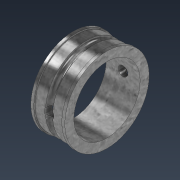
# Autodesk Inventor part: Łożysko wału korbowego 2
Saved by Autodesk Inventor 2022 (Build 260153000, 153)
## iProperties
Created: 2023-05-20
Part Number: Łożysko wału korbowego 2
Material: Generic
Document SubType Name: Modeling
Designer: wikto
Density: 1 g/cm^3
Appearance: Steel Galvanized
Author: wikto
Autodesk Inventor part; units mm, degrees
ref_plane "YZ Plane" through (0, 0, 0) normal (1, 0, 0) x (0, 1, 0)
ref_plane "XZ Plane" through (0, 0, 0) normal (0, 1, 0) x (-1, 0, 0)
ref_plane "XY Plane" through (0, 0, 0) normal (0, 0, 1) x (1, 0, 0)
sketch "Sketch1" plane through (0, 0, 0) normal (0, 0, 1) x (1, 0, 0)
  line L0 (-50, 0) -> (50, 0)
  line L1 (-14.086, 27.5) -> (-14.086, 35)
  line L2 (-14.086, 27.5) -> (14.086, 27.5)
  line L3 (14.086, 27.5) -> (14.086, 35)
  arc A0 (-3, 34) -> (3, 34) centre (0, 34) ccw
  line L4 (-14.086, 35) -> (-11.586, 35)
  line L5 (-11.586, 35) -> (-11.586, 34)
  line L6 (-11.586, 34) -> (-3, 34)
  line L7 (14.086, 35) -> (11.586, 35)
  line L8 (11.586, 35) -> (11.586, 34)
  line L9 (11.586, 34) -> (3, 34)
  point P0 (0, 0)
  point P1 (0, 0)
  point P2 (0, 27.5)
  dimension "d0" = 100
  dimension "d1" = 3
  dimension "d3" = 55
  dimension "d4" = 28.172
  dimension "d9" = 2.5
  dimension "d10" = 1
  dimension "d11" = 70
  constraints: 20 end point, 5 perpendicular, 4 horizontal, 2 equal length, 2 horizontal alignment, 2 midpoint, 2 point on circle, 2 vertical alignment, 1 centre point, 1 coincident, 1 vertical
  measures "d0" distance of L0.start L0.end
  measures "d1" radius of A0
  measures "d3" diameter of L2 L0
  measures "d4" distance between parallel lines of L3 L1
  measures "d9" distance of L3.end L7.end
  measures "d10" distance between parallel lines of L6 L4
  measures "d11" diameter of L7 L0
revolve "Revolution1" add sketch "Sketch1" angle 360 about axis through (-50, 0, 0) along (1, 0, 0)
sketch "Sketch2" plane through (0, 0, 0) normal (0, 0, 1) x (1, 0, 0)
  circle A0 centre (0, 0) radius 4
  dimension "d6" = 8
  constraints: 1 centre point, 1 coincident
  measures "d6" diameter of A0
extrude "Extrusion1" cut sketch "Sketch2" along normal through all both and the other way through all
body "Solid1"
